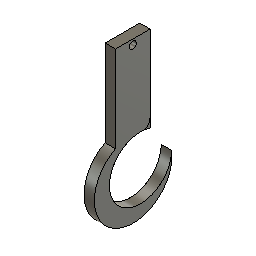
GUINCHO (Autodesk Fusion 360 design; units mm, degrees)
part number: 2026-06-04-15-32-03-257
Autodesk Fusion 360 part; units mm, degrees
sketch "Esboço1" plane through (0, 0, 0) normal (1, 0, 0) x (0, 0, -1)
  line L0 (0, 0) -> (10, 0)
  line L1 (10, 0) -> (10, -25)
  line L2 (0, 0) -> (0, -25)
  line L3 (0, -25) -> (10, -25)
  circle A0 centre (5, -1.5) radius 1
  arc A1 (0, -25) -> (10.229, -25) centre (5.1145, -34.985) ccw
  line L4 (10.229, -25) -> (10, -25)
  dimension "d1" = 10
  dimension "d2" = 25
  constraint coincident L0.start L2.start
  constraint horizontal L0
  constraint perpendicular L0 L1
  constraint perpendicular L0 L2
  constraint perpendicular L1 L3
  constraint perpendicular L1 L4
  measures "d1" distance of L0.start L0.end
  measures "d2" distance of L0.end L1.end
extrude "Extrusão1" add sketch "Esboço1" along normal blind 3 makes body 1
extrude "Extrusão2" add sketch "Esboço1" along normal blind 3 separate body makes body 2
hole "Furo3" at (3, -33.3851, -7.2358) direction (-1, 0, 0) diameter 18 depth 20 tip angle 118 bodies 1 2
fillet "Arredondamento2" radius 2 1 edges at (1.5, -24.8201, -10) on bodies 2
hole "Furo1" [rolled back] hole depth 19 hole diameter 20 tip angle 118
fillet "Arredondamento1" [rolled back] radius 0.5
hole "Furo2" [rolled back] hole depth 12 hole diameter 16 tip angle 118
moveface "MoverFace1" [rolled back]
